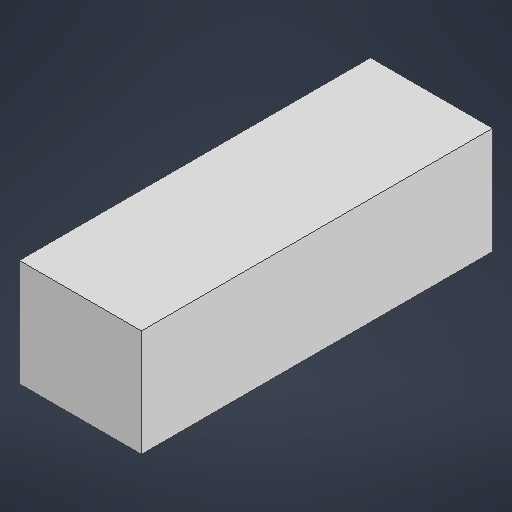
# Autodesk Inventor part: Batteryyyy
Saved by Autodesk Inventor 2026.1 (Build 301233000, 233)
## iProperties
Created: 2026-07-05
Part Number: Batteryyyy
Material: Generic
Document SubType Name: Modeling
Designer: Kasi Pusuluri
Density: 1 g/cm^3
Appearance: Default
Author: Kasi Pusuluri
Autodesk Inventor part; units mm, degrees
ref_plane "YZ Plane" through (0, 0, 0) normal (1, 0, 0) x (0, 1, 0)
ref_plane "XZ Plane" through (0, 0, 0) normal (0, 1, 0) x (-1, 0, 0)
ref_plane "XY Plane" through (0, 0, 0) normal (0, 0, 1) x (1, 0, 0)
sketch "Sketch2" plane through (0, 0, 0) normal (0, 1, 0) x (-1, 0, 0)
  line L0 (0, 0) -> (16, 0)
  line L1 (16, 0) -> (16, -46)
  line L2 (16, -46) -> (0, -46)
  line L3 (0, -46) -> (0, 0)
  dimension "d2" = 46
  dimension "d3" = 16
  constraints: 8 end point, 2 parallel, 1 horizontal, 1 perpendicular
  measures "d2" distance of L0.end L1.end
  measures "d3" distance of L1.end L2.end
extrude "Extrusion1" add sketch "Sketch2" along normal blind 14
body "Solid1"
